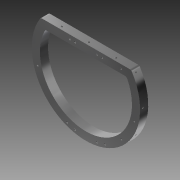
# Autodesk Inventor part: Middle Plate
Saved by Autodesk Inventor 2015 (Build 190159000, 159)
## iProperties
Created: 2016-02-17
Part Number: Middle Plate
Material: ABS Plastic
Document SubType Name: Modeling
Designer: 23902
Density: 1.06 g/cm^3
Appearance: Smooth - White
Author: 23902
Autodesk Inventor part; units mm, degrees
ref_plane "YZ Plane" through (0, 0, 0) normal (1, 0, 0) x (0, 1, 0)
ref_plane "XZ Plane" through (0, 0, 0) normal (0, 1, 0) x (-1, 0, 0)
ref_plane "XY Plane" through (0, 0, 0) normal (0, 0, 1) x (1, 0, 0)
sketch "Sketch1" plane through (0, 0, 0) normal (0, 1, 0) x (-1, 0, 0)
  line L0 (5.2, 50) -> (5.2, 45.6)
  line L1 (5.2, 45.6) -> (-5.2, 45.6)
  line L2 (-5.2, 45.6) -> (-5.2, 50)
  arc A0 (2.5852, 50) -> (-0.0053, 51.8093) centre (0.0011, 49.0593) ccw
  arc A1 (-0.0053, 51.8093) -> (-2.583, 50) centre (0.0011, 49.0593) ccw
  line L3 (-5.2, 50) -> (-2.583, 50)
  line L4 (5.2, 50) -> (2.5852, 50)
  line L5 (-0.0053, 51.8093) -> (0, 55)
  line L6 (-42.9966, 53.2175) -> (-40.7966, 49.407)
  line L7 (-48.4092, 52.1817) -> (-50, 54.9476)
  arc A2 (-45.2611, 51.9101) -> (-48.4092, 52.1817) centre (-47.0286, 49.8033) ccw
  arc A3 (-48.4092, 52.1817) -> (-49.7369, 49.326) centre (-47.0286, 49.8033) ccw
  line L8 (-52.0033, 48.0175) -> (-49.7369, 49.326)
  line L9 (-49.8033, 44.207) -> (-52.0033, 48.0175)
  line L10 (-40.7966, 49.407) -> (-49.8033, 44.207)
  line L11 (-42.9966, 53.2175) -> (-45.2611, 51.9101)
  line L12 (-79.6724, 52.0033) -> (-75.8619, 49.8033)
  line L13 (-83.842, 48.4) -> (-86.6025, 50)
  arc A4 (-80.9798, 49.7389) -> (-83.842, 48.4) centre (-81.4572, 47.0306) ccw
  arc A5 (-83.842, 48.4) -> (-83.5639, 45.2631) centre (-81.4572, 47.0306) ccw
  line L14 (-84.8724, 42.9967) -> (-83.5639, 45.2631)
  line L15 (-81.0619, 40.7967) -> (-84.8724, 42.9967)
  line L16 (-75.8619, 49.8033) -> (-81.0619, 40.7967)
  line L17 (-79.6724, 52.0033) -> (-80.9798, 49.7389)
  line L18 (-95, 5.2) -> (-90.6, 5.2)
  line L19 (-96.8093, -0.0053) -> (-100, 0)
  arc A6 (-95, 2.5852) -> (-96.8093, -0.0053) centre (-94.0593, 0.0011) ccw
  arc A7 (-96.8093, -0.0053) -> (-95, -2.583) centre (-94.0593, 0.0011) ccw
  line L20 (-95, -5.2) -> (-95, -2.583)
  line L21 (-90.6, -5.2) -> (-95, -5.2)
  line L22 (-90.6, 5.2) -> (-90.6, -5.2)
  line L23 (-95, 5.2) -> (-95, 2.5852)
  line L24 (-84.8724, -42.9967) -> (-81.0619, -40.7967)
  line L25 (-83.8366, -48.4093) -> (-86.6025, -50)
  arc A8 (-83.565, -45.2611) -> (-83.8366, -48.4093) centre (-81.4583, -47.0287) ccw
  arc A9 (-83.8366, -48.4093) -> (-80.9809, -49.7369) centre (-81.4583, -47.0287) ccw
  line L26 (-79.6724, -52.0033) -> (-80.9809, -49.7369)
  line L27 (-75.8619, -49.8033) -> (-79.6724, -52.0033)
  line L28 (-81.0619, -40.7967) -> (-75.8619, -49.8033)
  line L29 (-84.8724, -42.9967) -> (-83.565, -45.2611)
  line L30 (-52.0033, -79.6724) -> (-49.8033, -75.8619)
  line L31 (-48.4, -83.842) -> (-50, -86.6025)
  arc A10 (-49.7389, -80.9798) -> (-48.4, -83.842) centre (-47.0306, -81.4572) ccw
  arc A11 (-48.4, -83.842) -> (-45.2631, -83.5639) centre (-47.0306, -81.4572) ccw
  line L32 (-42.9967, -84.8724) -> (-45.2631, -83.5639)
  line L33 (-40.7967, -81.0619) -> (-42.9967, -84.8724)
  line L34 (-49.8033, -75.8619) -> (-40.7967, -81.0619)
  line L35 (-52.0033, -79.6724) -> (-49.7389, -80.9798)
  line L36 (-5.2, -95) -> (-5.2, -90.6)
  line L37 (0.0053, -96.8093) -> (0, -100)
  arc A12 (-2.5852, -95) -> (0.0053, -96.8093) centre (-0.0011, -94.0593) ccw
  arc A13 (0.0053, -96.8093) -> (2.583, -95) centre (-0.0011, -94.0593) ccw
  line L38 (5.2, -95) -> (2.583, -95)
  line L39 (5.2, -90.6) -> (5.2, -95)
  line L40 (-5.2, -90.6) -> (5.2, -90.6)
  line L41 (-5.2, -95) -> (-2.5852, -95)
  line L42 (42.9967, -84.8724) -> (40.7967, -81.0619)
  line L43 (48.4093, -83.8366) -> (50, -86.6025)
  arc A14 (45.2611, -83.565) -> (48.4093, -83.8366) centre (47.0287, -81.4583) ccw
  arc A15 (48.4093, -83.8366) -> (49.7369, -80.9809) centre (47.0287, -81.4583) ccw
  line L44 (52.0033, -79.6724) -> (49.7369, -80.9809)
  line L45 (49.8033, -75.8619) -> (52.0033, -79.6724)
  line L46 (40.7967, -81.0619) -> (49.8033, -75.8619)
  line L47 (42.9967, -84.8724) -> (45.2611, -83.565)
  line L48 (79.6724, -52.0033) -> (75.8619, -49.8033)
  line L49 (83.842, -48.4) -> (86.6025, -50)
  arc A16 (80.9798, -49.7389) -> (83.842, -48.4) centre (81.4572, -47.0306) ccw
  arc A17 (83.842, -48.4) -> (83.5639, -45.2631) centre (81.4572, -47.0306) ccw
  line L50 (84.8724, -42.9967) -> (83.5639, -45.2631)
  line L51 (81.0619, -40.7967) -> (84.8724, -42.9967)
  line L52 (75.8619, -49.8033) -> (81.0619, -40.7967)
  line L53 (79.6724, -52.0033) -> (80.9798, -49.7389)
  line L54 (95, -5.2) -> (90.6, -5.2)
  line L55 (96.8093, 0.0053) -> (100, 0)
  arc A18 (95, -2.5852) -> (96.8093, 0.0053) centre (94.0593, -0.0011) ccw
  arc A19 (96.8093, 0.0053) -> (95, 2.583) centre (94.0593, -0.0011) ccw
  line L56 (95, 5.2) -> (95, 2.583)
  line L57 (90.6, 5.2) -> (95, 5.2)
  line L58 (90.6, -5.2) -> (90.6, 5.2)
  line L59 (95, -5.2) -> (95, -2.5852)
  line L60 (84.8724, 42.9967) -> (81.0619, 40.7967)
  line L61 (83.8366, 48.4093) -> (86.6025, 50)
  arc A20 (83.565, 45.2611) -> (83.8366, 48.4093) centre (81.4583, 47.0287) ccw
  arc A21 (83.8366, 48.4093) -> (80.9809, 49.7369) centre (81.4583, 47.0287) ccw
  line L62 (79.6724, 52.0033) -> (80.9809, 49.7369)
  line L63 (75.8619, 49.8033) -> (79.6724, 52.0033)
  line L64 (81.0619, 40.7967) -> (75.8619, 49.8033)
  line L65 (84.8724, 42.9967) -> (83.565, 45.2611)
  line L66 (52.0033, 48.067) -> (49.8033, 44.2565)
  line L67 (48.4, 52.2366) -> (50, 54.9971)
  arc A22 (49.7389, 49.3744) -> (48.4, 52.2366) centre (47.0306, 49.8518) ccw
  arc A23 (48.4, 52.2366) -> (45.2631, 51.9585) centre (47.0306, 49.8518) ccw
  line L68 (42.9967, 53.267) -> (45.2631, 51.9585)
  line L69 (40.7967, 49.4565) -> (42.9967, 53.267)
  line L70 (49.8033, 44.2565) -> (40.7967, 49.4565)
  line L71 (52.0033, 48.067) -> (49.7389, 49.3744)
  line L72 (0, 55) -> (80.7775, 55)
  line L73 (0, 55) -> (-80.7775, 55)
  line L74 (0, 40) -> (71.9375, 40)
  line L75 (0, 40) -> (-71.9375, 40)
  arc A24 (-76.4336, 37.1875) -> (76.4336, 37.1875) centre (0, 0) ccw
  arc A25 (-85.0289, 52.6316) -> (85.0289, 52.6316) centre (0, 0) ccw
  arc A26 (85.0289, 52.6316) -> (80.7775, 55) centre (80.7775, 50) ccw
  arc A27 (76.4336, 37.1875) -> (71.9375, 40) centre (71.9375, 35) ccw
  arc A28 (-71.9375, 40) -> (-76.4336, 37.1875) centre (-71.9375, 35) ccw
  arc A29 (-80.7775, 55) -> (-85.0289, 52.6316) centre (-80.7775, 50) ccw
  line L76 (0, 55) -> (0, 47.5)
  circle A30 centre (-30, 47.5) radius 1.6
  circle A31 centre (30, 47.5) radius 1.6
  circle A32 centre (35, -88.3176) radius 1.6
  circle A33 centre (-35, -88.3176) radius 1.6
  circle A34 centre (-89.3481, -23.9408) radius 1.6
  circle A35 centre (89.3481, -23.9408) radius 1.6
  circle A36 centre (-20, 47.5) radius 1.6
  circle A37 centre (20, 47.5) radius 1.6
  circle A38 centre (-20, -92.5) radius 1.6
  circle A39 centre (20, -92.5) radius 1.6
  circle A40 centre (-65.4074, -65.4074) radius 1.6
  line L77 (-71.9375, 40) -> (-64.9375, 40)
  circle A41 centre (-64.9375, 47.5) radius 1.6
  point P0 (83.5165, 55)
  point P1 (-83.5165, 55)
  point P2 (75, 40)
  point P3 (-75, 40)
  dimension "d4" = 360
  dimension "d23" = 5
  dimension "d25" = 7.5
  dimension "d53" = 3.2
  dimension "d54" = 3.2
  constraints: 156 end point, 64 point on circle, 42 centre point, 14 coincident, 8 tangent, 7 point on line, 3 equal radius, 2 horizontal, 1 vertical, 145 other
  measures "d23" radius of A26
  measures "d25" distance of L72.start L76.end
  measures "d53" diameter of A36
  measures "d54" diameter of A37
extrude "Extrusion1" add sketch "Sketch1" along normal blind 15 contours L72 A26 A25 A29 L73 | A0 L5 L76
sketch "Sketch3" plane through (0, 0, 0) normal (0, -1, 0) x (1, 0, 0)
  line L0 (-40.7967, 49.4565) -> (-49.8033, 44.2565) projected
  line L1 (-49.8033, 44.2565) -> (-52.0033, 48.067) projected
  line L2 (-52.0033, 48.067) -> (-49.7389, 49.3744) projected
  arc A0 (-45.2631, 51.9585) -> (-49.7389, 49.3744) centre (-47.0306, 49.8518) ccw projected
  line L3 (-45.2631, 51.9585) -> (-42.9967, 53.267) projected
  line L4 (-42.9967, 53.267) -> (-40.7967, 49.4565) projected
  line L5 (-75.8619, 49.8033) -> (-81.0619, 40.7967) projected
  line L6 (-81.0619, 40.7967) -> (-84.8724, 42.9967) projected
  line L7 (-84.8724, 42.9967) -> (-83.565, 45.2611) projected
  arc A1 (-80.9809, 49.7369) -> (-83.565, 45.2611) centre (-81.4583, 47.0287) ccw projected
  line L8 (-80.9809, 49.7369) -> (-79.6724, 52.0033) projected
  line L9 (-79.6724, 52.0033) -> (-75.8619, 49.8033) projected
  line L10 (-90.6, 5.2) -> (-90.6, -5.2) projected
  line L11 (-90.6, -5.2) -> (-95, -5.2) projected
  line L12 (-95, -5.2) -> (-95, -2.5852) projected
  arc A2 (-95, 2.583) -> (-95, -2.5852) centre (-94.0593, -0.0011) ccw projected
  line L13 (-95, 2.583) -> (-95, 5.2) projected
  line L14 (-95, 5.2) -> (-90.6, 5.2) projected
  line L15 (-81.0619, -40.7967) -> (-75.8619, -49.8033) projected
  line L16 (-75.8619, -49.8033) -> (-79.6724, -52.0033) projected
  line L17 (-79.6724, -52.0033) -> (-80.9798, -49.7389) projected
  arc A3 (-83.5639, -45.2631) -> (-80.9798, -49.7389) centre (-81.4572, -47.0306) ccw projected
  line L18 (-83.5639, -45.2631) -> (-84.8724, -42.9967) projected
  line L19 (-84.8724, -42.9967) -> (-81.0619, -40.7967) projected
  line L20 (-49.8033, -75.8619) -> (-40.7967, -81.0619) projected
  line L21 (-40.7967, -81.0619) -> (-42.9967, -84.8724) projected
  line L22 (-42.9967, -84.8724) -> (-45.2611, -83.565) projected
  arc A4 (-49.7369, -80.9809) -> (-45.2611, -83.565) centre (-47.0287, -81.4583) ccw projected
  line L23 (-49.7369, -80.9809) -> (-52.0033, -79.6724) projected
  line L24 (-52.0033, -79.6724) -> (-49.8033, -75.8619) projected
  line L25 (-5.2, -90.6) -> (5.2, -90.6) projected
  line L26 (5.2, -90.6) -> (5.2, -95) projected
  line L27 (5.2, -95) -> (2.5852, -95) projected
  arc A5 (-2.583, -95) -> (2.5852, -95) centre (0.0011, -94.0593) ccw projected
  line L28 (-2.583, -95) -> (-5.2, -95) projected
  line L29 (-5.2, -95) -> (-5.2, -90.6) projected
  line L30 (40.7967, -81.0619) -> (49.8033, -75.8619) projected
  line L31 (49.8033, -75.8619) -> (52.0033, -79.6724) projected
  line L32 (52.0033, -79.6724) -> (49.7389, -80.9798) projected
  arc A6 (45.2631, -83.5639) -> (49.7389, -80.9798) centre (47.0306, -81.4572) ccw projected
  line L33 (45.2631, -83.5639) -> (42.9967, -84.8724) projected
  line L34 (42.9967, -84.8724) -> (40.7967, -81.0619) projected
  line L35 (75.8619, -49.8033) -> (81.0619, -40.7967) projected
  line L36 (81.0619, -40.7967) -> (84.8724, -42.9967) projected
  line L37 (84.8724, -42.9967) -> (83.565, -45.2611) projected
  arc A7 (80.9809, -49.7369) -> (83.565, -45.2611) centre (81.4583, -47.0287) ccw projected
  line L38 (80.9809, -49.7369) -> (79.6724, -52.0033) projected
  line L39 (79.6724, -52.0033) -> (75.8619, -49.8033) projected
  line L40 (90.6, -5.2) -> (90.6, 5.2) projected
  line L41 (90.6, 5.2) -> (95, 5.2) projected
  line L42 (95, 5.2) -> (95, 2.5852) projected
  arc A8 (95, -2.583) -> (95, 2.5852) centre (94.0593, 0.0011) ccw projected
  line L43 (95, -2.583) -> (95, -5.2) projected
  line L44 (95, -5.2) -> (90.6, -5.2) projected
  line L45 (81.0619, 40.7967) -> (75.8619, 49.8033) projected
  line L46 (75.8619, 49.8033) -> (79.6724, 52.0033) projected
  line L47 (79.6724, 52.0033) -> (80.9798, 49.7389) projected
  arc A9 (83.5639, 45.2631) -> (80.9798, 49.7389) centre (81.4572, 47.0306) ccw projected
  line L48 (83.5639, 45.2631) -> (84.8724, 42.9967) projected
  line L49 (84.8724, 42.9967) -> (81.0619, 40.7967) projected
  line L50 (49.8033, 44.207) -> (40.7966, 49.407) projected
  line L51 (40.7966, 49.407) -> (42.9966, 53.2175) projected
  line L52 (42.9966, 53.2175) -> (45.2611, 51.9101) projected
  arc A10 (49.7369, 49.326) -> (45.2611, 51.9101) centre (47.0286, 49.8033) ccw projected
  line L53 (49.7369, 49.326) -> (52.0033, 48.0175) projected
  line L54 (52.0033, 48.0175) -> (49.8033, 44.207) projected
  line L55 (5.2, 45.6) -> (-5.2, 45.6) projected
  line L56 (-5.2, 45.6) -> (-5.2, 50) projected
  line L57 (-5.2, 50) -> (-2.5852, 50) projected
  arc A11 (2.583, 50) -> (-2.5852, 50) centre (-0.0011, 49.0593) ccw projected
  line L58 (2.583, 50) -> (5.2, 50) projected
  line L59 (5.2, 50) -> (5.2, 45.6) projected
  point P0 (0, 0)
extrude "Extrusion2" add sketch "Sketch3" against normal blind 2
sketch "Sketch4" plane through (-5.2, 15, 45.6) normal (0, 0, 1) x (1, 0, 0)
  line L0 (0, 0) -> (10.4, 0) projected
  line L1 (5.2, 0) -> (5.2, -9.5)
  circle A0 centre (5.2, -9.5) radius 1.5
  point P0 (5.2, -15)
  dimension "d30" = 9.5
  dimension "d31" = 3
  constraints: 2 end point, 1 centre point, 1 coincident, 1 midpoint, 1 vertical
  measures "d30" distance of L1.start L1.end
  measures "d31" diameter of A0
extrude "Extrusion3" cut sketch "Sketch4" along normal through all
sketch "Sketch5" plane through (-40.7967, 2, 49.4565) normal (-0.5, 0, 0.8660254) x (0.8660254, 0, 0.5)
  line L0 (-10.4, 13) -> (0, 13) projected
  line L1 (-5.2, 13) -> (-5.2, 3.5)
  circle A0 centre (-5.2, 3.5) radius 1.5
  point P0 (10.6027, -2)
  dimension "d34" = 9.5
  dimension "d35" = 3
  constraints: 2 end point, 1 centre point, 1 coincident, 1 midpoint, 1 vertical
  measures "d34" distance of L1.start L1.end
  measures "d35" diameter of A0
extrude "Extrusion4" cut sketch "Sketch5" along normal through all
sketch "Sketch6" plane through (49.8033, 2, 44.207) normal (0.5, 0, 0.8660254) x (0.8660254, 0, -0.5)
  line L0 (-10.4, 13) -> (0, 13) projected
  line L1 (-5.2, 13) -> (-5.2, 3.5)
  circle A0 centre (-5.2, 3.5) radius 1.5
  point P0 (-21.0274, -2)
  dimension "d38" = 9.5
  dimension "d39" = 3
  constraints: 2 end point, 1 centre point, 1 coincident, 1 midpoint, 1 vertical
  measures "d38" distance of L1.start L1.end
  measures "d39" diameter of A0
extrude "Extrusion5" cut sketch "Sketch6" along normal through all
sketch "Sketch7" plane through (81.0619, 2, 40.7967) normal (0.8660254, 0, 0.5) x (0.5, 0, -0.8660254)
  line L0 (-10.4, 13) -> (0, 13) projected
  line L1 (-5.2, 13) -> (-5.2, 3.5)
  circle A0 centre (-5.2, 3.5) radius 1.5
  point P0 (-5.2, -2)
  dimension "d42" = 9.5
  dimension "d43" = 3
  constraints: 2 end point, 1 centre point, 1 coincident, 1 midpoint, 1 vertical
  measures "d42" distance of L1.start L1.end
  measures "d43" diameter of A0
extrude "Extrusion6" cut sketch "Sketch7" along normal through all
pattern_circular "Circular Pattern1" count 9 over 240 about axis through (0, -10, 0) along (0, 1, 0) of "Extrusion6"
body "Solid1"
